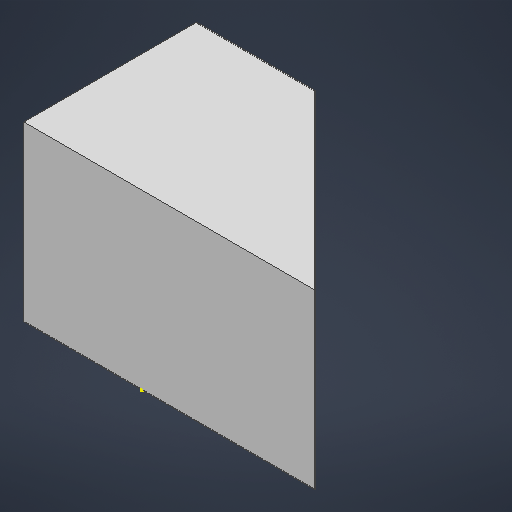
# Autodesk Inventor part: Cajon_ascensor_mejorsita
Saved by Autodesk Inventor 2026.2 (Build 302298010, 298A)
## iProperties
Created: 2026-04-28
Part Number: Cajon_ascensor_mejorsita
Material: Genérico
Document SubType Name: Modeling
Designer: agusb
Density: 1 g/cm^3
Appearance: Valor por defecto
Author: agusb
Autodesk Inventor part; units mm, degrees
ref_plane "YZ Plane" through (0, 0, 0) normal (1, 0, 0) x (0, 1, 0)
ref_plane "XZ Plane" through (0, 0, 0) normal (0, 1, 0) x (-1, 0, 0)
ref_plane "XY Plane" through (0, 0, 0) normal (0, 0, 1) x (1, 0, 0)
sketch "Boceto1" plane through (0, 0, 0) normal (0, 1, 0) x (-1, 0, 0)
  line L0 (0, 0) -> (0, -350)
  line L1 (0, -350) -> (-350, 0)
  line L2 (-350, 0) -> (0, 0)
  dimension "d0" = 350
  dimension "d1" = 45
  constraints: 6 end point, 1 perpendicular, 1 vertical
  measures "d0" distance of L0.start L0.end
  measures "d1" angle of L0 L1
extrude "Extrusión1" add sketch "Boceto1" along normal blind 1
sketch "Boceto2" plane through (0, 1, 0) normal (0, 1, 0) x (1, 0, 0)
  line L0 (350, 0) -> (0, 350) projected
  line L1 (174.2929, 174.2929) -> (348.5858, 0)
  line L2 (0, 0) -> (350, 0) projected
  line L3 (174.2929, 174.2929) -> (420.7803, 174.2929) construction
  line L4 (348.5858, 1) -> (-0.0002, 1)
  line L5 (0, 350) -> (0, 0) projected
  line L6 (174.2929, 174.2929) -> (0, 348.5858)
  point P0 (347.5858, 1)
  point P1 (0, 1)
  dimension "d5" = 45
  dimension "d6" = 1
  dimension "d7" = 348.586
  constraints: 8 end point, 3 point on line, 1 equal length, 1 horizontal, 1 perpendicular
  measures "d5" angle of L1 L3
  measures "d6" distance of L1.end L4.start
  measures "d7" distance of L4.start L4.end
extrude "Extrusión2" add sketch "Boceto2" along normal blind 348 contours L2 L1 L6 L5 L0 | L2 L5 L4 L1
sketch "Boceto3" plane through (0, 349, 0) normal (0, 1, 0) x (1, 0, 0)
  line L0 (0, 350) -> (0, 0) projected
  line L1 (0, 0) -> (0, 350)
  line L2 (0, 0) -> (350, 0) projected
  line L3 (0, 350) -> (350, 0)
  line L4 (350, 0) -> (0, 0)
  constraints: 6 end point, 1 perpendicular, 1 vertical
extrude "Extrusión3" add sketch "Boceto3" along normal blind 1
sketch "Boceto4" plane through (0, 0, -350) normal (-1, 0, 0) x (0, 0, 1)
  point P0 (350, 0)
sketch "Boceto5" plane through (0, 0, -350) normal (-1, 0, 0) x (0, 0, 1)
  line L0 (0, 0) -> (0, 350) projected
  line L1 (350, 0) -> (0, 0)
  line L2 (0, 0) -> (0, 350)
  line L3 (0, 350) -> (350, 350)
  line L4 (350, 350) -> (350, 0)
  line L5 (349, 1) -> (1.4142, 1) projected
  line L6 (1.4142, 1) -> (1.4142, 349) projected
  line L7 (349, 1) -> (1.4142, 1)
  line L8 (1.4142, 1) -> (1.4142, 349)
  line L9 (1.4142, 349) -> (349, 349)
  line L10 (349, 349) -> (349, 1)
  constraints: 16 end point, 4 parallel, 2 horizontal, 2 perpendicular
extrude "Extrusión4" add sketch "Boceto5" along normal blind 240
